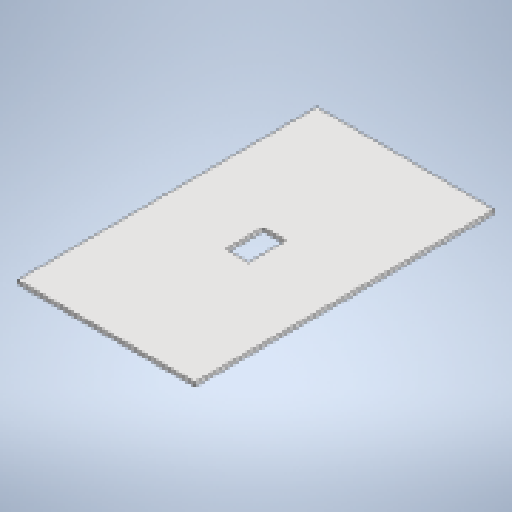
# Autodesk Inventor part: TapaBaterias
Saved by Autodesk Inventor 2024 (Build 280153000, 153)
## iProperties
Created: 2024-07-14
Part Number: TapaBaterias
Material: Genérico
Document SubType Name: Modeling
Designer: sergi
Density: 1 g/cm^3
Appearance: Valor por defecto
Author: sergi
Autodesk Inventor part; units mm, degrees
ref_plane "YZ Plane" through (0, 0, 0) normal (1, 0, 0) x (0, 1, 0)
ref_plane "XZ Plane" through (0, 0, 0) normal (0, 1, 0) x (-1, 0, 0)
ref_plane "XY Plane" through (0, 0, 0) normal (0, 0, 1) x (1, 0, 0)
sketch "Boceto1" plane through (0, 0, 0) normal (0, 1, 0) x (-1, 0, 0)
  line L0 (-24.25, -40.9) -> (24.25, -40.9)
  line L1 (24.25, -40.9) -> (24.25, 40.9)
  line L2 (24.25, 40.9) -> (-24.25, 40.9)
  line L3 (-24.25, 40.9) -> (-24.25, -40.9)
  line L4 (-24.25, -40.9) -> (24.25, 40.9) construction
  line L5 (24.25, -40.9) -> (-24.25, 40.9) construction
  point P0 (0, 0)
  dimension "d0" = 48.5
  dimension "d1" = 81.8
  constraints: 12 end point, 2 midpoint, 2 parallel, 1 horizontal, 1 perpendicular
  measures "d0" distance of L2.end L1.end
  measures "d1" distance of L1.end L0.end
extrude "Extrusión1" add sketch "Boceto1" along normal blind 1
sketch "Boceto2" plane through (0, 1, 0) normal (0, 1, 0) x (1, 0, 0)
  line L0 (3.1, 5.1) -> (-3.1, 5.1)
  line L1 (-3.1, 5.1) -> (-3.1, -5.1)
  line L2 (-3.1, -5.1) -> (3.1, -5.1)
  line L3 (3.1, -5.1) -> (3.1, 5.1)
  line L4 (3.1, 5.1) -> (-3.1, -5.1) construction
  line L5 (-3.1, 5.1) -> (3.1, -5.1) construction
  point P0 (0, 0)
  dimension "d4" = 6.2
  dimension "d5" = 10.2
  constraints: 12 end point, 2 midpoint, 2 parallel, 1 horizontal, 1 perpendicular
  measures "d4" distance of L2.end L1.end
  measures "d5" distance of L1.end L0.end
extrude "Extrusión2" cut sketch "Boceto2" against normal blind 1
sketch "Boceto3" plane through (0, 0, 0) normal (0, -1, 0) x (1, 0, 0)
  line L0 (-22.25, -40.9) -> (-17.25, -40.9) projected
  line L1 (-17.25, -38.9) -> (-22.25, -38.9) projected
  line L2 (-17.25, -40.9) -> (-17.25, -38.9) projected
  line L3 (-22.25, 29.1) -> (-22.25, -40.9) projected
  line L4 (-22.25, 29.1) -> (-24.25, 29.1) projected
  line L5 (22.25, 38.9) -> (-24.25, 38.9) projected
  line L6 (-24.25, 29.1) -> (32.137, 29.1)
  line L7 (32.137, 29.1) -> (32.137, 38.9)
  line L8 (32.137, 38.9) -> (-24.25, 38.9)
  line L9 (-24.25, 38.9) -> (-24.25, 29.1)
  line L10 (-17.25, -40.9) -> (-22.25, -40.9)
  line L11 (-22.25, -40.9) -> (-22.25, -38.9)
  line L12 (-22.25, -38.9) -> (-17.25, -38.9)
  line L13 (-17.25, -38.9) -> (-17.25, -40.9)
  point P0 (0, 0)
  constraints: 16 end point, 4 parallel, 2 horizontal, 2 perpendicular, 1 point on line
extrude "Extrusión3" add sketch "Boceto3" along normal blind 4.3 contours L3 L1 L2 L0
sketch "Boceto4" plane through (0, 0, 0) normal (0, -1, 0) x (1, 0, 0)
  line L0 (-24.25, 29.1) -> (-22.25, 29.1) projected
  line L1 (-24.25, -40.9) -> (-24.25, 40.9) projected
  line L2 (-22.25, 29.1) -> (-24.25, 29.1)
  line L3 (-24.25, 29.1) -> (-24.25, 40.9)
  line L4 (-24.25, 40.9) -> (-22.25, 40.9)
  line L5 (-22.25, 40.9) -> (-22.25, 29.1)
  line L6 (-24.25, 38.9) -> (22.25, 38.9) projected
  point P0 (0, 0)
  point P1 (-22.25, 38.9)
  constraints: 8 end point, 2 parallel, 1 horizontal, 1 perpendicular
extrude "Extrusión4" add sketch "Boceto4" along normal blind 8.85 contours L1 L6 L5 L0
sketch "Boceto5" plane through (0, 0, 0) normal (0, -1, 0) x (1, 0, 0)
  line L0 (24.25, -40.9) -> (24.25, 40.9) projected
  line L1 (24.25, 40.9) -> (-24.25, 40.9) projected
  line L2 (22.25, 38.9) -> (22.25, 29.1) projected
  line L3 (-24.25, 38.9) -> (22.25, 38.9) projected
  line L4 (22.25, 29.1) -> (-17.25, 29.1) projected
  line L5 (22.25, 38.9) -> (24.25, 38.9)
  line L6 (24.25, 38.9) -> (24.25, 29.1)
  line L7 (24.25, 29.1) -> (22.25, 29.1)
  line L8 (22.25, 29.1) -> (22.25, 38.9)
  point P0 (0, 0)
  constraints: 8 end point, 2 parallel, 1 horizontal, 1 perpendicular, 1 point on line
extrude "Extrusión5" add sketch "Boceto5" along normal blind 3.1
